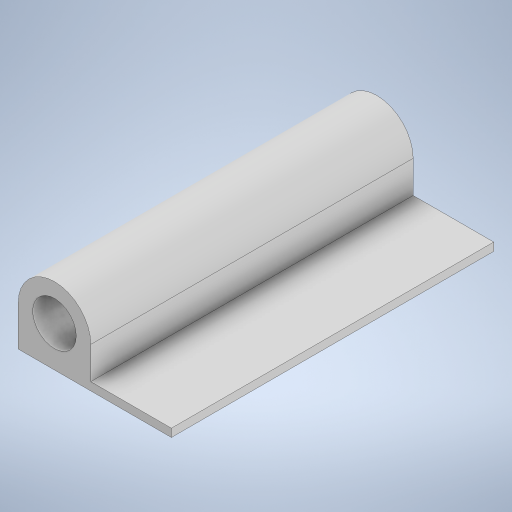
# Autodesk Inventor part: LI0017-LATCH BARREL
Saved by Autodesk Inventor 2023 (Build 270158000, 158)
## iProperties
Created: 2023-05-10
Part Number: LI0017-LATCH BARREL
Material: Generic
Document SubType Name: Modeling
Designer: Louis
Density: 1 g/cm^3
Appearance: Default
Author: Louis
Autodesk Inventor part; units mm, degrees
ref_plane "YZ Plane" through (0, 0, 0) normal (1, 0, 0) x (0, 1, 0)
ref_plane "XZ Plane" through (0, 0, 0) normal (0, 1, 0) x (-1, 0, 0)
ref_plane "XY Plane" through (0, 0, 0) normal (0, 0, 1) x (1, 0, 0)
sketch "Sketch1" plane through (0, 0, 0) normal (0, 0, 1) x (1, 0, 0)
  line L0 (9, 0) -> (28, 0)
  line L1 (28, 0) -> (28, 1)
  line L2 (28, 1) -> (9, 1)
  line L3 (9, 1) -> (18, 1)
  line L4 (18, 1) -> (18, 5)
  line L5 (18, 5) -> (9, 5)
  line L6 (9, 5) -> (9, 1)
  circle A0 centre (13.5, 5) radius 4.5
  circle A1 centre (13.5, 5) radius 2.5
  line L7 (9, 1) -> (9, 0)
  point P0 (0, 0)
  point P1 (28, 0.5)
  point P2 (18, 1)
  point P3 (11.4384, 1)
  point P4 (15.5616, 1)
  dimension "d1" = 1
  dimension "d2" = 5
  dimension "d3" = 5
  dimension "d4" = 2
  dimension "d5" = 10
  dimension "d11" = 9
  constraints: 16 end point, 3 parallel, 3 perpendicular, 2 horizontal, 2 midpoint, 1 centre point, 1 coincident, 3 other
  measures "d1" distance between parallel lines of L0 L2
  measures "d2" distance between parallel lines of L0 L5
  measures "d3" diameter of A1
  measures "d5" distance from line of point (28, 0.5) L4
  measures "d11" distance of point (0, 0) L0.start
extrude "Extrusion1" add sketch "Sketch1" along normal blind 40 contours L7 L2 A0 L1 L0 | L6 A0 L2 | A0 L5 A1 L2 | L2 A0 | A0 L5 A1 | L2 A0 L4
thicken "Thicken1" operation cut thickness 0.2 both sides no extend neighbours no toward (0.9870503, -0.1604113, 0) faces at (15.9676, 4.599, 26.6667)
body "Solid1"
